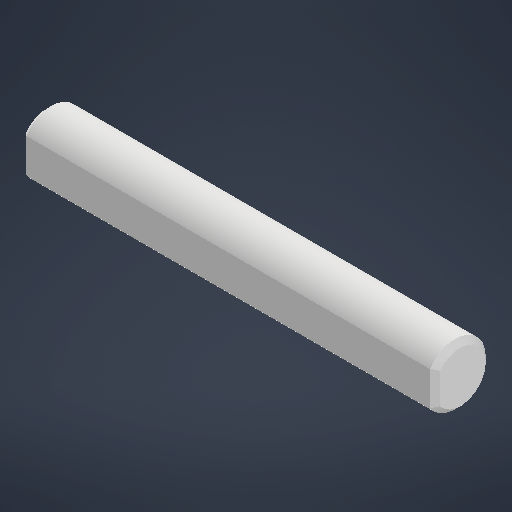
# Autodesk Inventor part: Ø6x40Shaft_Modified
Saved by Autodesk Inventor 2026 (Build 300175050, 175E)
## iProperties
Created: 2026-05-02
Part Number: Ø6x40Shaft_Modified
Material: Generic
Document SubType Name: Modeling
Designer: frede
Density: 1 g/cm^3
Appearance: Default
Author: frede
Autodesk Inventor part; units mm, degrees
ref_plane "YZ Plane" through (0, 0, 0) normal (1, 0, 0) x (0, 1, 0)
ref_plane "XZ Plane" through (0, 0, 0) normal (0, 1, 0) x (-1, 0, 0)
ref_plane "XY Plane" through (0, 0, 0) normal (0, 0, 1) x (1, 0, 0)
sketch "Sketch1" plane through (0, 0, 0) normal (1, 0, 0) x (0, 1, 0)
  circle A0 centre (0, 0) radius 2.95
  line L0 (1.6432, 2.45) -> (-1.6432, 2.45)
  dimension "d0" = 5.9
  dimension "d1" = 0.5
  constraints: 2 end point, 2 point on circle, 1 centre point, 1 coincident, 1 horizontal
  measures "d0" diameter of A0
  measures "d1" distance edge to line of A0 L0
extrude "Extrusion1" add sketch "Sketch1" along normal blind 40 contours A0 L0 picked at (0.5577, 0.5097)
chamfer "Chamfer1" distance 0.5 angle 45 4 edges at (0, 0, -2.95) (0, 0, 2.45) (40, 0, -2.95) (40, 0, 2.45)
body "Solid1"
